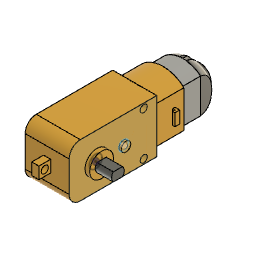
moteur (Autodesk Fusion 360 design; units mm, degrees)
Autodesk Fusion 360 part; units mm, degrees
note: some values were not read from the file. Chosen so that the rebuilt part matches the saved one: which face or edge a step refers to. Set by a fixed rule: which sketch regions a step uses.
sketch "Esquisse1" plane through (0, 0, 0) normal (0, 0, 1) x (1, 0, 0)
  line L0 (0, -11.2) -> (9.3, -11.2)
  line L1 (0, -11.2) -> (-9.3, -11.2)
  line L2 (-9.3, -11.2) -> (-9.3, 25.8)
  line L3 (9.3, -11.2) -> (9.3, 25.8)
  line L4 (9.3, 25.8) -> (-9.3, 25.8)
  dimension "d4" = 9.3
  dimension "d5" = 37
  constraint perpendicular L1 L2
  constraint perpendicular L0 L3
  constraint perpendicular L2 L4
  measures "d4" distance of L0.start L0.end
  measures "d5" distance of L1.end L2.end
extrude "Extrusion1" add sketch "Esquisse1" along normal blind 11.2 and the other way blind 11.2 makes body 1
fillet "Congé1" radius 4.7 1 edges at (0, -11.2, 11.2) on bodies 1
fillet "Congé2" radius 4.7 1 edges at (0, -11.2, -11.2) on bodies 1
sketch "Esquisse2" plane through (9.3, 0, 0) normal (1, 0, 0) x (0, 1, 0)
  arc A0 (-11.2, -6.5) -> (-6.5, -11.2) centre (-6.5, -6.5) ccw
  line L0 (-6.5, -11.2) -> (25.8, -11.2)
  line L1 (25.8, -11.2) -> (25.8, 11.2)
  line L2 (25.8, 11.2) -> (-6.5, 11.2)
  arc A1 (-6.5, 11.2) -> (-11.2, 6.5) centre (-6.5, 6.5) ccw
  line L3 (-11.2, 6.5) -> (-11.2, -6.5)
  circle A2 centre (20.3, 9.2) radius 1.5
  dimension "d12" = 3
  dimension "d13" = 20.3
  dimension "d14" = 9.2
  measures "d12" diameter of A2
  measures "d13" horizontal distance of origin A2.centre
  measures "d14" vertical distance of origin A2.centre
hole "Perçage1" at (9.3, 20.3, 9.2) direction (-1, 0, 0) diameter 3 depth 20 tip angle 118 bodies 1
mirror "Symétrie miroir1" about plane through (0, 0, 0) normal (0, 0, 1) of "Perçage1"
sketch "Esquisse3" plane through (0, 25.8, 0) normal (0, 1, 0) x (-1, 0, 0)
  line L0 (9.3, -11.2) -> (9.3, 11.2)
  line L1 (9.3, 11.2) -> (-9.3, 11.2)
  line L2 (-9.3, 11.2) -> (-9.3, -11.2)
  line L3 (-9.3, -11.2) -> (9.3, -11.2)
  line L4 (8.8, 7.75) -> (8.8, -7.85)
  line L5 (-8.8, 7.75) -> (-8.8, -7.85)
  line L6 (-8.8, -7.85) -> (8.8, -7.85)
  line L7 (-8.8, 7.75) -> (8.8, 7.75)
  ellipse E0 centre (0, 0) end of major axis (0, 11.2) minor radius 12.32
  line L8 (0, -11.2) -> (0, 11.2)
  line L9 (12.32, 0) -> (-12.32, 0)
  line L10 (8.8, 7.75) -> (8.8, 8)
  line L11 (-8.8, 7.75) -> (-8.8, 8)
  dimension "d24" = 24.64
  dimension "d25" = 17.6
  dimension "d26" = 15.6
  constraint perpendicular L4 L6
  constraint perpendicular L4 L7
  constraint coincident E0.centre origin
  constraint perpendicular L1 L8
  constraint coincident E0 L8.start
  constraint coincident E0 L8.end
  constraint coincident E0 L9.start
  constraint coincident E0 L9.end
  constraint perpendicular L7 L10
  constraint perpendicular L7 L11
  measures "d25" distance of L5.start L4.start
  measures "d26" distance of L4.start L4.end
extrude "Extrusion2" add sketch "Esquisse3" along normal blind 12 contours L6 E0 L8 | L6 E0 L8 | L4 L6 E0 L8 L9 | L5 L6 E0 L8 L9 | L4 L7 L8 L9 | L5 L7 L8 L9 | L7 E0 L8 L10 | L7 E0 L8 L11 bodies 1
sketch "Esquisse4" plane through (0, 37.8, 0) normal (0, 1, 0) x (-1, 0, 0)
  line L0 (8.8, -7.8384) -> (8.8, 7.8384)
  ellipse E0 centre (0, 0) end of major axis (-12.32, 0) minor radius 11.2 (8.8, 7.8384) -> (-8.8, 7.8384) ccw
  line L1 (-8.8, 7.8384) -> (-8.8, -7.8384)
  ellipse E1 centre (0, 0) end of major axis (-12.32, 0) minor radius 11.2 (-8.8, -7.8384) -> (8.8, -7.8384) ccw
  line L2 (-7.5, 7.3) -> (7.5, 7.3)
  line L3 (7.5, 7.3) -> (7.5, -7.3)
  line L4 (7.5, -7.3) -> (-7.5, -7.3)
  line L5 (-7.5, -7.3) -> (-7.5, 7.3)
  ellipse E2 centre (0, 0) end of major axis (0, 10) minor radius 11
  line L6 (0, -10) -> (0, 10)
  line L7 (11, 0) -> (-11, 0)
  line L8 (7.7326, 7.3) -> (-7.7631, 7.3)
  line L9 (-7.5789, -7.3) -> (8.8, -7.3)
  point P0 (-7.5, 7.3)
  point P1 (-7.5, 0)
  dimension "d29" = 15
  dimension "d30" = 14.6
  dimension "d31" = 0
  constraint horizontal L2
  constraint vertical L3
  constraint horizontal L4
  constraint vertical L5
  constraint coincident P0 L2.start
  constraint midpoint L5 P1
  constraint coincident E0.centre E1.centre
  constraint perpendicular L2 L6
  constraint coincident E2 L6.start
  constraint coincident E2 L6.end
  constraint coincident E2 L7.start
  constraint coincident E2 L7.end
  constraint perpendicular L5 L8
  constraint coincident L0 L9.end
  constraint perpendicular L0 L9
  measures "d29" distance of P0 L2.end
  measures "d30" distance of P0 L4.end
  measures "d31" distance of E0.centre P1
extrude "Extrusion3" add sketch "Esquisse4" along normal blind 8.3 separate body contours L4 E2 L6 L9 | L4 E2 L6 L9 | L3 L4 L6 L7 L9 | L2 L3 L6 L7 L8 | L4 L5 L6 L7 L9 | L2 L5 L6 L7 L8 | L2 E2 L6 L8 | L2 E2 L6 L8 makes body 2
sketch "Esquisse5" plane through (0, 0, 0) normal (1, 0, 0) x (0, 1, 0)
  line L0 (51.3865, 10.0214) -> (45.9865, 10.0214)
  line L1 (45.9865, 10.0214) -> (45.9865, 4.6214)
  line L2 (45.9865, 4.6214) -> (51.3865, 4.6214)
  line L3 (51.3865, 4.6214) -> (51.3865, 10.0214)
  circle A0 centre (45.9865, 4.6214) radius 5.3
  dimension "d34" = 5.4
  dimension "d35" = 5.4
  dimension "d36" = 10.6
  constraint horizontal L0
  constraint vertical L1
  constraint horizontal L2
  constraint vertical L3
  constraint coincident L1.end L2.start
  measures "d34" distance of L0.start L0.end
  measures "d35" distance of L0.start L2.end
  measures "d36" diameter of A0
extrude "Extrusion4" add 1 faces at (0, 46.1, -3.3333) along direction (0, 1, 0) blind 5.3 separate body on bodies 2 makes body 3
revolve "Révolution1" add sketch "Esquisse5" angle 360 about axis through (0, 1.75, 0) along (0, 1, 0) separate body contours L0 L1 L2 L3 A0 makes body 4
scale "Echelle1" factors (1.1, 1.01, 1) about (0, 51.2865, 4.6214) bodies 4
combine "Combiner1" operation cut target body 3 tool bodies 4
extrude "Extrusion5" cut 1 faces at (-0.4586, 51.4, 3.3072) along direction (0, -1, 0) blind 0.1 on bodies 3 bodies 3
sketch "Esquisse6" plane through (0, 46.1, 0) normal (0, 1, 0) x (-1, 0, 0)
  line L0 (7.5179, -7.3) -> (7.5, -7.3)
  line L1 (7.5, -7.3) -> (7.5, 7.3)
  line L2 (7.5, 7.3) -> (7.5179, 7.3)
  ellipse E0 centre (0, 0) end of major axis (-11, 0) minor radius 10 (7.5179, 7.3) -> (-7.5179, 7.3) ccw
  line L3 (-7.5179, 7.3) -> (-7.5, 7.3)
  line L4 (-7.5, 7.3) -> (-7.5, -7.3)
  line L5 (-7.5, -7.3) -> (-7.5179, -7.3)
  ellipse E1 centre (0, 0) end of major axis (-11, 0) minor radius 10 (-7.5179, -7.3) -> (7.5179, -7.3) ccw
  circle A0 centre (0, 8.5) radius 1.5
  line L6 (0, 10) -> (1.5, 10)
  line L7 (1.5, 10) -> (1.5, 11.5)
  line L8 (1.5, 11.5) -> (0, 11.5)
  line L9 (0, 11.5) -> (0, 10)
  line L10 (0, 10) -> (-1.5, 10)
  line L11 (-1.5, 10) -> (-1.5, 8.5)
  line L12 (-1.5, 8.5) -> (0, 8.5)
  line L13 (0, 8.5) -> (0, 10)
  line L14 (-1.5, 10) -> (0, 10)
  line L15 (0, 10) -> (0, 11.5)
  line L16 (0, 11.5) -> (-1.5, 11.5)
  line L17 (-1.5, 11.5) -> (-1.5, 10)
  line L18 (0, 8.5) -> (1.5, 8.5)
  line L19 (1.5, 8.5) -> (1.5, 10)
  line L20 (1.5, 10) -> (0, 10)
  line L21 (0, 10) -> (0, 8.5)
  dimension "d45" = 3
  dimension "d47" = 1.5
  dimension "d48" = 1.5
  dimension "d49" = 1.5
  constraint horizontal L6
  constraint vertical L7
  constraint horizontal L8
  constraint vertical L9
  constraint horizontal L10
  constraint vertical L11
  constraint horizontal L12
  constraint vertical L13
  constraint horizontal L14
  constraint vertical L15
  constraint horizontal L16
  constraint vertical L17
  constraint horizontal L18
  constraint vertical L19
  constraint horizontal L20
  constraint vertical L21
  measures "d45" diameter of A0
  measures "d47" distance of L6.start L6.end
  measures "d48" distance of L6.start L8.end
  measures "d49" distance of L6.start A0.centre
extrude "Extrusion6" cut sketch "Esquisse6" along normal blind 6 contours A0 L12 L18 bodies 3
extrude "Extrusion7" cut sketch "Esquisse6" along normal blind 6 contours A0 L12 L13 L21 | A0 L13 L18 L21 bodies 3
extrude "Extrusion8" cut sketch "Esquisse6" along normal blind 6 contours E0 A0 L19 bodies 3
extrude "Extrusion9" cut sketch "Esquisse6" along normal blind 6 contours E0 A0 L11 bodies 3
mirror "Symétrie miroir2" about plane through (0, 0, 0) normal (0, 0, 1) of "Extrusion6", "Extrusion7", "Extrusion8", "Extrusion9"
cylinder "CylinderPrimitive1" add diameter 9.6 height 2 placed x (1, 0, 0) y (0, 0, -1) z (0, 1, 0) at (0, 51.3, 0) bodies 3
cylinder "CylinderPrimitive2" add diameter 1.9 height 1 placed x (1, 0, 0) y (0, 0, -1) z (0, 1, 0) at (0, 53.3, 0) bodies 3
sketch "Esquisse10" plane through (-8.8, 0, 0) normal (-1, 0, 0) x (0, -1, 0)
  line L0 (-25.8, -7.8384) -> (-25.8, 7.8384)
  line L1 (-25.8, 7.8384) -> (-37.8, 7.8384)
  line L2 (-37.8, 7.8384) -> (-37.8, -7.8384)
  line L3 (-37.8, -7.8384) -> (-25.8, -7.8384)
  line L4 (-32, 2.55) -> (-34, 2.55)
  line L5 (-34, 2.55) -> (-34, -2.55)
  line L6 (-34, -2.55) -> (-32, -2.55)
  line L7 (-32, -2.55) -> (-32, 2.55)
  dimension "d67" = 2
  dimension "d68" = 5.1
  dimension "d69" = 32
  dimension "d70" = 2.55
  constraint horizontal L4
  constraint vertical L5
  constraint horizontal L6
  constraint vertical L7
  measures "d67" distance of L4.start L4.end
  measures "d68" distance of L4.start L6.end
  measures "d69" distance of origin L7
  measures "d70" distance of origin L4
extrude "Extrusion10" add sketch "Esquisse10" along normal blind 2 contours L4 L5 L6 L7 bodies 1
sketch "Esquisse11" plane through (0, 0, 2.55) normal (0, 0, 1) x (-1, 0, 0)
  line L0 (8.8, -32) -> (8.8, -34)
  line L1 (8.8, -34) -> (10.8, -34)
  line L2 (10.8, -34) -> (10.8, -32)
  line L3 (10.8, -32) -> (8.8, -32)
  line L4 (8.8, -32) -> (9.8, -32)
  line L5 (9.8, -32) -> (9.8, -33)
  line L6 (9.8, -33) -> (8.8, -33)
  line L7 (8.8, -33) -> (8.8, -32)
  constraint horizontal L4
  constraint vertical L5
  constraint horizontal L6
  constraint vertical L7
  constraint coincident L0.start L3.end
extrude "Extrusion11" cut sketch "Esquisse11" against normal blind 5.2 contours L0 L3 L4 L5 L6 L7 bodies 1
mirror "Symétrie miroir3" about plane through (0, 0, 0) normal (1, 0, 0) of "Extrusion10", "Extrusion11"
sketch "Esquisse12" plane through (9.3, 0, 0) normal (1, 0, 0) x (0, 1, 0)
  circle A0 centre (20.3, -9.2) radius 1.5
  circle A1 centre (20.3, 9.2) radius 1.5
  arc A2 (-11.2, -6.5) -> (-6.5, -11.2) centre (-6.5, -6.5) ccw
  line L0 (-6.5, -11.2) -> (25.8, -11.2)
  line L1 (25.8, -11.2) -> (25.8, 11.2)
  line L2 (25.8, 11.2) -> (-6.5, 11.2)
  arc A3 (-6.5, 11.2) -> (-11.2, 6.5) centre (-6.5, 6.5) ccw
  line L3 (-11.2, 6.5) -> (-11.2, -6.5)
  circle A4 centre (11.8, 0) radius 2
  circle A5 centre (0, 0) radius 2.675
  dimension "d76" = 4
  dimension "d77" = 11.8
  dimension "d89" = 5.35
  constraint coincident A5.centre origin
  measures "d76" diameter of A4
  measures "d77" distance of A5.centre A4.centre
  measures "d89" diameter of A5
extrude "Extrusion14" add sketch "Esquisse12" along normal blind 0.5 separate body contours A5 makes body 5
extrude "Extrusion12" add sketch "Esquisse12" along normal blind 1 contours A4 bodies 1
sketch "Esquisse13" plane through (0, -11.2, 0) normal (0, -1, 0) x (1, 0, 0)
  line L0 (-9.3, -6.5) -> (9.3, -6.5)
  line L1 (9.3, -6.5) -> (9.3, 6.5)
  line L2 (9.3, 6.5) -> (-9.3, 6.5)
  line L3 (-9.3, 6.5) -> (-9.3, -6.5)
  line L4 (-1.5, 2.5) -> (1.5, 2.5)
  line L5 (1.5, 2.5) -> (1.5, -2.5)
  line L6 (1.5, -2.5) -> (-1.5, -2.5)
  line L7 (-1.5, -2.5) -> (-1.5, 2.5)
  dimension "d80" = 3
  dimension "d81" = 5
  dimension "d82" = 2.5
  dimension "d83" = 1.5
  constraint horizontal L4
  constraint vertical L5
  constraint horizontal L6
  constraint vertical L7
  measures "d80" distance of L4.start L4.end
  measures "d81" distance of L4.start L6.end
  measures "d82" distance of origin L4
  measures "d83" distance of origin L7
extrude "Extrusion13" add sketch "Esquisse13" along normal blind 5 contours L4 L5 L6 L7 bodies 1
hole "Perçage2" at (1.5, -13.7, 0) direction (-1, 0, 0) diameter 3 depth 20 tip angle 118 bodies 1
sketch "Esquisse14" plane through (9.8, 0, 0) normal (1, 0, 0) x (0, 1, 0)
  circle A0 centre (0, 0) radius 2.675
  line L0 (0, 0) -> (2.675, 0)
  line L1 (2.675, 0) -> (2.675, -1.85)
  line L2 (2.675, -1.85) -> (0, -1.85)
  line L3 (0, -1.85) -> (0, 0)
  line L4 (0, -1.85) -> (-2.675, -1.85)
  line L5 (-2.675, -1.85) -> (-2.675, 0)
  line L6 (-2.675, 0) -> (0, 0)
  line L7 (0, 0) -> (0, -1.85)
  line L8 (-2.675, 0) -> (0, 0)
  line L9 (0, 0) -> (0, 1.85)
  line L10 (0, 1.85) -> (-2.675, 1.85)
  line L11 (-2.675, 1.85) -> (-2.675, 0)
  line L12 (0, 1.85) -> (2.675, 1.85)
  line L13 (2.675, 1.85) -> (2.675, 0)
  line L14 (2.675, 0) -> (0, 0)
  line L15 (0, 0) -> (0, 1.85)
  dimension "d92" = 2.675
  dimension "d93" = 1.85
  dimension "d94" = 2.675
  dimension "d95" = 1.85
  constraint horizontal L0
  constraint vertical L1
  constraint horizontal L2
  constraint vertical L3
  constraint coincident A0.centre L0.start
  constraint horizontal L4
  constraint vertical L5
  constraint horizontal L6
  constraint vertical L7
  constraint horizontal L8
  constraint vertical L9
  constraint horizontal L10
  constraint vertical L11
  constraint horizontal L12
  constraint vertical L13
  constraint horizontal L14
  constraint vertical L15
  measures "d92" distance of A0.centre L0.end
  measures "d93" distance of A0.centre L2.end
  measures "d94" distance of L2.end L4.end
  measures "d95" distance of L5.end L10.end
extrude "Extrusion15" add sketch "Esquisse14" along normal blind 8.9 contours A0 L0 L9 L12 L14 L15 | A0 L0 L2 L3 L7 L14 | A0 L3 L4 L6 L7 L8 | A0 L6 L8 L9 L10 L15 bodies 5
cylinder "CylinderPrimitive3" add diameter 10 height 2 placed x (0, 0, -1) y (0, 1, 0) z (1, 0, 0) at (9.8, 0, 0) separate body makes body 6
combine "Combiner2" operation cut target body 6 tool bodies 5 keep tools
named bodies: "Corps plastique", "Extrémité métallique", "Corps métallique", "Arbre de transmission", "Rondelle"
